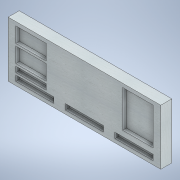
# Autodesk Inventor part: Base
Saved by Autodesk Inventor 2022.4 (Build 264492010, 492A)
## iProperties
Created: 2023-02-14
Part Number: Base
Material: Genérico
Document SubType Name: Modeling
Designer: wob19
Density: 1 g/cm^3
Appearance: Valor por defecto
Author: wob19
Autodesk Inventor part; units mm, degrees
ref_plane "YZ Plane" through (0, 0, 0) normal (1, 0, 0) x (0, 1, 0)
ref_plane "XZ Plane" through (0, 0, 0) normal (0, 1, 0) x (-1, 0, 0)
ref_plane "XY Plane" through (0, 0, 0) normal (0, 0, 1) x (1, 0, 0)
sketch "Boceto1" plane through (0, 0, 0) normal (0, 0, 1) x (1, 0, 0)
  line L0 (-275, -100) -> (275, -100)
  line L1 (275, -100) -> (275, 100)
  line L2 (275, 100) -> (-275, 100)
  line L3 (-275, 100) -> (-275, -100)
  line L4 (-275, -100) -> (275, 100) construction
  line L5 (275, -100) -> (-275, 100) construction
  point P0 (0, 0)
  dimension "ancho" = 550
  dimension "alto" = 200
  constraints: 12 end point, 2 midpoint, 2 parallel, 1 horizontal, 1 perpendicular
  measures "ancho" distance of L2.end L1.end
  measures "alto" distance of L1.end L0.end
extrude "Extrusión1" add sketch "Boceto1" along normal blind 40
sketch "Boceto2" plane through (0, 0, 40) normal (0, 0, 1) x (1, 0, 0)
  line L0 (247.5, -86.6667) -> (110, -86.6667)
  line L1 (110, -86.6667) -> (110, -66.6667)
  line L2 (110, -66.6667) -> (247.5, -66.6667)
  line L3 (247.5, -66.6667) -> (247.5, -86.6667)
  line L4 (275, -100) -> (275, 100) projected
  line L5 (-110, -86.6667) -> (-247.5, -86.6667)
  line L6 (-247.5, -86.6667) -> (-247.5, -66.6667)
  line L7 (-247.5, -66.6667) -> (-110, -66.6667)
  line L8 (-110, -66.6667) -> (-110, -86.6667)
  line L9 (-275, 100) -> (-275, -100) projected
  line L10 (-275, -100) -> (275, -100) projected
  line L11 (68.75, -86.6667) -> (-68.75, -86.6667)
  line L12 (-68.75, -86.6667) -> (-68.75, -66.6667)
  line L13 (-68.75, -66.6667) -> (68.75, -66.6667)
  line L14 (68.75, -66.6667) -> (68.75, -86.6667)
  line L15 (275, 100) -> (-275, 100) projected
  line L16 (247.5, 86.6667) -> (137.5, 86.6667)
  line L17 (137.5, 86.6667) -> (137.5, -46.6667)
  line L18 (137.5, -46.6667) -> (247.5, -46.6667)
  line L19 (247.5, -46.6667) -> (247.5, 86.6667)
  line L20 (-247.5, 86.6667) -> (-137.5, 86.6667)
  line L21 (-137.5, 86.6667) -> (-137.5, 31.6667)
  line L22 (-137.5, 31.6667) -> (-247.5, 31.6667)
  line L23 (-247.5, 31.6667) -> (-247.5, 86.6667)
  line L24 (-247.5, 23.8235) -> (-137.5, 23.8235)
  line L25 (-137.5, 23.8235) -> (-137.5, -31.1765)
  line L26 (-137.5, -31.1765) -> (-247.5, -31.1765)
  line L27 (-247.5, -31.1765) -> (-247.5, 23.8235)
  line L28 (-247.5, -59.0196) -> (-137.5, -59.0196)
  line L29 (-137.5, -59.0196) -> (-137.5, -39.0196)
  line L30 (-137.5, -39.0196) -> (-247.5, -39.0196)
  line L31 (-247.5, -39.0196) -> (-247.5, -59.0196)
  point P0 (0, 0)
  dimension "d4" = 137.5
  dimension "d5" = 20
  dimension "d6" = 27.5
  dimension "d7" = 137.5
  dimension "d8" = 20
  dimension "d9" = 27.5
  dimension "d10" = 13.3333
  dimension "d11" = 13.3333
  dimension "d12" = 137.5
  dimension "d13" = 41.25
  dimension "d14" = 41.25
  dimension "d15" = 20
  dimension "d17" = 110
  dimension "d18" = 133.3333
  dimension "d19" = 27.5
  dimension "d20" = 13.3333
  dimension "d21" = 110
  dimension "d22" = 55
  dimension "d23" = 27.5
  dimension "d24" = 13.3333
  dimension "d25" = 110
  dimension "d26" = 55
  dimension "d27" = 27.5
  dimension "d28" = 7.8431
  dimension "d29" = 110
  dimension "d30" = 20
  dimension "d31" = 7.8431
  dimension "d32" = 7.6471
  constraints: 56 end point, 14 parallel, 7 horizontal, 7 perpendicular
  measures "d4" distance of L1.end L2.end
  measures "d5" distance of L2.end L0.start
  measures "d6" distance between parallel lines of L4 L3
  measures "d7" distance of L6.end L7.end
  measures "d8" distance of L5.end L6.end
  measures "d9" distance between parallel lines of L9 L6
  measures "d10" distance between parallel lines of L10 L0
  measures "d11" distance between parallel lines of L10 L5
  measures "d12" distance of L12.end L13.end
  measures "d13" distance between parallel lines of L1 L14
  measures "d14" distance between parallel lines of L8 L12
  measures "d15" distance of L13.end L11.start
  measures "d17" distance of L18.end L17.end
  measures "d18" distance of L17.end L16.end
  measures "d19" distance between parallel lines of L4 L19
  measures "d20" distance between parallel lines of L15 L16
  measures "d21" distance of L21.end L22.end
  measures "d22" distance of L20.end L21.end
  measures "d23" distance between parallel lines of L9 L23
  measures "d24" distance between parallel lines of L15 L20
  measures "d25" distance of L25.end L26.end
  measures "d26" distance of L24.end L25.end
  measures "d27" distance between parallel lines of L9 L27
  measures "d28" distance between parallel lines of L22 L24
  measures "d29" distance of L28.start L28.end
  measures "d30" distance of L30.end L28.start
  measures "d31" distance between parallel lines of L26 L30
  measures "d32" distance between parallel lines of L28 L7
extrude "Extrusión2" cut sketch "Boceto2" against normal blind 13.3333 contours L0 L1 L2 L3 | L5 L6 L7 L8 | L11 L12 L13 L14 | L19 L18 L17 L16 | L20 L21 L22 L23 | L24 L25 L26 L27 | L31 L30 L29 L28
sketch "Boceto3" plane through (0, 0, 0) normal (0, 0, -1) x (-1, 0, 0)
  circle A0 centre (255, -33.3333) radius 10
  circle A1 centre (255, 33.3333) radius 10
  circle A2 centre (-255, 33.3333) radius 10
  circle A3 centre (-255, -33.3333) radius 10
  line L0 (275, 100) -> (275, -100) projected
  line L1 (275, -100) -> (-275, -100) projected
  line L2 (-275, 100) -> (275, 100) projected
  line L3 (-275, -100) -> (-275, 100) projected
  point P0 (0, 0)
  dimension "d35" = 20
  dimension "d36" = 20
  dimension "d37" = 20
  dimension "d38" = 20
  dimension "d39" = 20
  dimension "d40" = 66.6667
  dimension "d41" = 20
  dimension "d42" = 66.6667
  dimension "d43" = 20
  dimension "d44" = 66.6667
  dimension "d45" = 20
  dimension "d46" = 66.6667
  constraints: 4 centre point
  measures "d35" diameter of A0
  measures "d36" diameter of A1
  measures "d37" diameter of A3
  measures "d38" diameter of A2
  measures "d39" distance from line of L0 A0.centre
  measures "d40" distance from line of L1 A0.centre
  measures "d41" distance from line of L0 A1.centre
  measures "d42" distance from line of L2 A1.centre
  measures "d43" distance from line of L3 A3.centre
  measures "d44" distance from line of L1 A3.centre
  measures "d45" distance from line of L3 A2.centre
  measures "d46" distance from line of L2 A2.centre
extrude "Extrusión3" cut sketch "Boceto3" against normal blind 13.3333 contours A0 | A1 | A2 | A3
equation "\"d4\" = 0.25 * ancho"
equation "\"d5\" = 0.1 * alto"
equation "\"d6\" = 0.05 * ancho"
equation "\"d7\" = d4"
equation "\"d8\" = d5"
equation "\"d9\" = d6"
equation "\"d10\" = 0.0666667 * alto"
equation "\"d11\" = 0.0666667 * alto"
equation "\"d12\" = d4"
equation "\"d13\" = d14"
equation "\"d15\" = d5"
equation "\"d17\" = 0.2 * ancho"
equation "\"d18\" = 0.666667 * alto"
equation "\"d19\" = d6"
equation "\"d20\" = d10"
equation "\"d21\" = 0.2 * ancho"
equation "\"d22\" = 0.1 * ancho"
equation "\"d23\" = d9"
equation "\"d24\" = d11"
equation "\"d25\" = d21"
equation "\"d26\" = d22"
equation "\"d27\" = d23"
equation "\"d28\" = 0.0392157 * alto"
equation "\"d29\" = d21"
equation "\"d30\" = d5"
equation "\"d31\" = d28"
equation "\"d33\" = 0.333333 * grosor"
equation "\"d35\" = 0.5 * grosor"
equation "\"d36\" = d35"
equation "\"d37\" = d35"
equation "\"d38\" = d35"
equation "\"d39\" = 0.5 * grosor"
equation "\"d40\" = 0.333333 * alto"
equation "\"d41\" = d39"
equation "\"d42\" = d40"
equation "\"d43\" = d39"
equation "\"d44\" = d40"
equation "\"d45\" = d39"
equation "\"d46\" = d40"
equation "\"d47\" = 0.333333 * grosor"
equation "\"grosor\" = 40"
